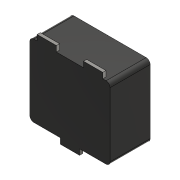
# Autodesk Inventor part: 20_018_SMD_VOLUME_G43A_R1
Saved by Autodesk Inventor 2021.2 (Build 252289000, 289)
## iProperties
Created: 2018-10-05
Part Number: 20_018_SMD_VOLUME_G43A_R1
Material: 一般
Document SubType Name: Modeling
Designer: student
Density: 1 g/cm^3
Appearance: 既定
Mass: 0.0527367 g
Surface Area: 1.11414 cm^2
Volume: 0.0527367 cm^3
Author: student
Autodesk Inventor part; units mm, degrees
ref_plane "YZ Plane" through (0, 0, 0) normal (1, 0, 0) x (0, 1, 0)
ref_plane "XZ Plane" through (0, 0, 0) normal (0, 1, 0) x (-1, 0, 0)
ref_plane "XY Plane" through (0, 0, 0) normal (0, 0, 1) x (1, 0, 0)
sketch "スケッチ1" plane through (0, 0, 0) normal (0, 1, 0) x (-1, 0, 0)
  line L0 (2.25, -2.25) -> (-2.25, -2.25)
  line L1 (-2.5, -2) -> (-2.5, 2)
  line L2 (-2.25, 2.25) -> (2.25, 2.25)
  line L3 (2.5, 2) -> (2.5, -2)
  line L4 (2.5, 0) -> (-2.5, 0) construction
  line L5 (0, -2.25) -> (0, 2.25) construction
  arc A0 (2.25, -2.25) -> (2.5, -2) centre (2.25, -2) ccw
  arc A1 (-2.5, -2) -> (-2.25, -2.25) centre (-2.25, -2) ccw
  arc A2 (-2.25, 2.25) -> (-2.5, 2) centre (-2.25, 2) ccw
  arc A3 (2.5, 2) -> (2.25, 2.25) centre (2.25, 2) ccw
  point P0 (0, 0)
  point P1 (2.5, -2.25)
  point P2 (-2.5, -2.25)
  point P3 (2.5, 2.25)
  dimension "d0" = 4.5
  dimension "d1" = 5
  dimension "d2" = 0.25
  constraints: 12 end point, 8 point on circle, 8 tangent, 6 midpoint, 6 point on line, 4 centre point, 3 equal radius, 2 parallel, 1 horizontal, 1 perpendicular
  measures "d0" distance of point (2.5, 2.25) point (2.5, -2.25)
  measures "d1" distance of point (2.5, -2.25) point (-2.5, -2.25)
  measures "d2" radius of A0
extrude "押し出し1" add sketch "スケッチ1" along normal blind 2.5
sketch "スケッチ2" plane through (0, 2.5, 0) normal (0, 1, 0) x (1, 0, 0)
  circle A0 centre (0, 0) radius 1.75
  circle A1 centre (0, 0) radius 2
  line L0 (1.5, 0) -> (0, 0) construction
  line L1 (0, 0) -> (0, 1.5) construction
  arc A2 (0.4, 1.4457) -> (-0.4, 1.4457) centre (0, 0) ccw
  arc A3 (1.4457, -0.4) -> (1.4457, 0.4) centre (0, 0) ccw
  arc A4 (0.4, 0.9) -> (0.9, 0.4) centre (0.9, 0.9) ccw
  line L2 (0.9, 0.4) -> (1.4457, 0.4)
  line L3 (0.4, 0.9) -> (0.4, 1.4457)
  arc A5 (-0.4, -1.4457) -> (0.4, -1.4457) centre (0, 0) ccw
  arc A6 (0.9, -0.4) -> (0.4, -0.9) centre (0.9, -0.9) ccw
  line L4 (0.9, -0.4) -> (1.4457, -0.4)
  line L5 (0.4, -0.9) -> (0.4, -1.4457)
  arc A7 (-1.4457, 0.4) -> (-1.4457, -0.4) centre (0, 0) ccw
  arc A8 (-0.9, 0.4) -> (-0.4, 0.9) centre (-0.9, 0.9) ccw
  line L6 (-0.9, 0.4) -> (-1.4457, 0.4)
  line L7 (-0.4, 0.9) -> (-0.4, 1.4457)
  line L8 (-0.4, -0.9) -> (-0.4, -1.4457)
  arc A9 (-0.4, -0.9) -> (-0.9, -0.4) centre (-0.9, -0.9) ccw
  line L9 (-0.9, -0.4) -> (-1.4457, -0.4)
  point P0 (0, -1.5)
  dimension "d5" = 0.8
  dimension "d6" = 0.8
  dimension "d7" = 1.5
  dimension "d8" = 0.5
  dimension "d9" = 3.5
  dimension "d10" = 4
  constraints: 20 end point, 19 point on circle, 16 symmetric about line, 10 centre point, 4 coincident, 2 horizontal, 2 tangent, 1 concentric, 1 perpendicular, 1 vertical, 5 other
  measures "d5" diameter of L3 L1
  measures "d6" diameter of L2 L0
  measures "d7" radius of A3
  measures "d8" radius of A4
  measures "d9" diameter of A0
  measures "d10" diameter of A1
extrude "押し出し2" cut sketch "スケッチ2" against normal blind 0.5
sketch "スケッチ3" plane through (0, 0, 0) normal (0, -1, 0) x (1, 0, 0)
  line L0 (2.25, -2.25) -> (-2.25, -2.25) construction
  line L1 (0.6, -2.25) -> (-0.6, -2.25)
  line L2 (-0.6, -2.25) -> (-0.6, -2.6)
  line L3 (-0.6, -2.6) -> (0.6, -2.6)
  line L4 (0.6, -2.6) -> (0.6, -2.25)
  line L5 (2.25, 2.25) -> (-2.25, 2.25) construction
  line L6 (-0.8452, 2.25) -> (-2.0452, 2.25)
  line L7 (-2.0452, 2.25) -> (-2.0452, 2.6)
  line L8 (-2.0452, 2.6) -> (-0.8452, 2.6)
  line L9 (-0.8452, 2.6) -> (-0.8452, 2.25)
  line L10 (0, 0) -> (0, 2.25) construction
  line L11 (0, 0) -> (-3.3171, 0) construction
  line L12 (0.8452, 2.25) -> (2.0452, 2.25)
  line L13 (2.0452, 2.25) -> (2.0452, 2.6)
  line L14 (2.0452, 2.6) -> (0.8452, 2.6)
  line L15 (0.8452, 2.6) -> (0.8452, 2.25)
  dimension "d14" = 5.2
  dimension "d15" = 1.2
  dimension "d16" = 1.2
  constraints: 28 end point, 4 parallel, 4 symmetric about line, 3 horizontal, 2 perpendicular, 2 point on line, 1 midpoint, 2 other
  measures "d14" diameter of L3 L11
  measures "d15" distance between parallel lines of L9 L7
  measures "d16" distance between parallel lines of L2 L4
extrude "押し出し3" add sketch "スケッチ3" against normal blind 0.2
